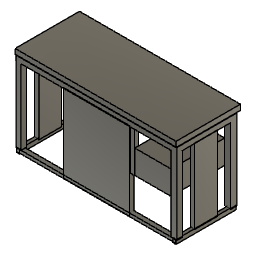
Project D2 (Autodesk Fusion 360 design; units mm, degrees)
Autodesk Fusion 360 part; units mm, degrees
sketch "Sketch1" plane through (0, 0, 0) normal (0, 1, 0) x (1, 0, 0)
  line L0 (-73.6158, -70.0302) -> (76.3842, -70.0302)
  line L1 (76.3842, -70.0302) -> (76.3842, -65.0302)
  line L2 (76.3842, -65.0302) -> (-73.6158, -65.0302)
  line L3 (-73.6158, -65.0302) -> (-73.6158, -70.0302)
  dimension "d1" = 150
  dimension "d2" = 5
  constraint horizontal L0
  constraint vertical L1
  constraint horizontal L2
  constraint vertical L3
  measures "d1" distance of L0.start L0.end
  measures "d2" distance of L0.start L2.end
extrude "Extrude1" add sketch "Sketch1" along normal blind 60 makes body 1
sketch "Sketch2" plane through (0, 0, 0) normal (0, 1, 0) x (1, 0, 0)
  line L0 (-71.4094, -65.6389) -> (74.5906, -65.6389)
  line L1 (74.5906, -65.6389) -> (74.5906, -70.6389)
  line L2 (74.5906, -70.6389) -> (-71.4094, -70.6389)
  line L3 (-71.4094, -70.6389) -> (-71.4094, -65.6389)
  dimension "d5" = 146
  dimension "d6" = 5
  constraint horizontal L0
  constraint vertical L1
  constraint horizontal L2
  constraint vertical L3
  measures "d5" distance of L0.start L0.end
  measures "d6" distance of L0.start L2.end
move_body "Move1" bodies 1 to x (1, 0, 0) y (0, 1, 0) z (0, 0, 1) at (0, 10, -40)
extrude "Extrude2" add sketch "Sketch2" along normal blind 56 separate body makes body 2
sketch "Sketch3" plane through (0, 0, 70.6389) normal (0, 0, 1) x (-1, 0, 0)
  line L0 (71.4094, 0) -> (-74.5906, 0)
  line L1 (-74.5906, 0) -> (-74.5906, -56)
  line L2 (-74.5906, -56) -> (71.4094, -56)
  line L3 (71.4094, -56) -> (71.4094, 0)
  line L4 (70, -51) -> (-70, -51)
  line L5 (-70, -51) -> (-70, -5)
  line L6 (-70, -5) -> (70, -5)
  line L7 (70, -5) -> (70, -51)
  dimension "d9" = 140
  dimension "d10" = 46
  constraint horizontal L4
  constraint vertical L5
  constraint horizontal L6
  constraint vertical L7
  measures "d9" distance of L4.start L4.end
  measures "d10" distance of L4.start L6.end
extrude "Extrude3" cut sketch "Sketch3" against normal blind 5 contours L4 L5 L6 L7 bodies 2
extrude "Extrude4" add 1 faces at (-71.4094, 18.6667, 68.9722) along direction (-1, 0, 0) blind 2 on bodies 2 bodies 2
sketch "Sketch4" plane through (0, 0, 0) normal (0, 1, 0) x (1, 0, 0)
move_body "Move2" bodies 1 to x (1, 0, 0) y (0, 1, 0) z (0, 0, 1) at (-149.7936, 0, 0)
extrude "Extrude5" add 1 faces at (-73.4094, 18.6667, 68.9722) along direction (-1, 0, 0) blind 2 on bodies 2 bodies 2
sketch "Sketch5" plane through (0, 0, 70.6389) normal (0, 0, 1) x (-1, 0, 0)
  line L0 (-70, -51) -> (-70, -5)
  line L1 (-70, -5) -> (70, -5)
  line L2 (70, -5) -> (70, -51)
  line L3 (70, -51) -> (-70, -51)
  line L4 (75.4094, 0) -> (-74.5906, 0)
  line L5 (-74.5906, 0) -> (-74.5906, -56)
  line L6 (-74.5906, -56) -> (75.4094, -56)
  line L7 (75.4094, -56) -> (75.4094, 0)
  line L8 (75.4094, -56) -> (70, -56)
  line L9 (70, -56) -> (70, -50)
  line L10 (70, -50) -> (75.4094, -50)
  line L11 (75.4094, -50) -> (75.4094, -56)
  constraint horizontal L8
  constraint vertical L9
  constraint horizontal L10
  constraint vertical L11
  constraint coincident L6.end L7.start
extrude "Extrude6" add sketch "Sketch5" along normal blind 60 contours L2 L6 L7 L8 L9 L10 L11 bodies 2
move_body "Move3" bodies 1 to x (1, 0, 0) y (0, 1, 0) z (0, 0, 1) at (-20, 0, 0)
sketch "Sketch6" plane through (0, 0, 70.6389) normal (0, 0, 1) x (-1, 0, 0)
  line L0 (70, -56) -> (70, -51)
  line L1 (70, -51) -> (-70, -51)
  line L2 (-70, -51) -> (-70, -5)
  line L3 (-70, -5) -> (70, -5)
  line L4 (70, -5) -> (70, -50)
  line L5 (70, -50) -> (75.4094, -50)
  line L6 (75.4094, -50) -> (75.4094, 0)
  line L7 (75.4094, 0) -> (-74.5906, 0)
  line L8 (-74.5906, 0) -> (-74.5906, -56)
  line L9 (-74.5906, -56) -> (70, -56)
  line L10 (-70, -56) -> (-74.4843, -56)
  line L11 (-74.4843, -56) -> (-74.4843, -51)
  line L12 (-74.4843, -51) -> (-70, -51)
  line L13 (-70, -51) -> (-70, -56)
  line L14 (-74.4843, -4.9712) -> (-70, -4.9712)
  line L15 (-70, -4.9712) -> (-70, 0)
  line L16 (-70, 0) -> (-74.4843, 0)
  line L17 (-74.4843, 0) -> (-74.4843, -4.9712)
  line L18 (70, 0) -> (75.4094, 0)
  line L19 (75.4094, 0) -> (75.4094, -5)
  line L20 (75.4094, -5) -> (70, -5)
  line L21 (70, -5) -> (70, 0)
  constraint horizontal L10
  constraint vertical L11
  constraint horizontal L12
  constraint vertical L13
  constraint coincident L9 L10.start
  constraint horizontal L14
  constraint vertical L15
  constraint horizontal L16
  constraint vertical L17
  constraint horizontal L18
  constraint vertical L19
  constraint horizontal L20
  constraint vertical L21
  constraint coincident L6 L19.end
  constraint coincident L7 L18.start
extrude "Extrude7" add sketch "Sketch6" along normal blind 70 contours L9 L10 L11 L12 L13 | L6 L7 L18 L19 L20 L21 | L7 L14 L15 L16 L17 bodies 2
extrude "Extrude8" add 1 faces at (-73.6062, 52.3333, 130.6389) along direction (0, 0, 1) blind 10 on bodies 2 bodies 2
sketch "Sketch7" plane through (0, 0, 0) normal (0, 1, 0) x (1, 0, 0)
  line L0 (-75.802, -140.9306) -> (74.198, -140.9306)
  line L1 (74.198, -140.9306) -> (74.198, -136.9306)
  line L2 (74.198, -136.9306) -> (-75.802, -136.9306)
  line L3 (-75.802, -136.9306) -> (-75.802, -140.9306)
  dimension "d23" = 150
  dimension "d24" = 4
  constraint horizontal L0
  constraint vertical L1
  constraint horizontal L2
  constraint vertical L3
  measures "d23" distance of L0.start L0.end
  measures "d24" distance of L0.start L2.end
extrude "Extrude9" add sketch "Sketch7" against normal blind 5 bodies 2
delete_face "DeleteFace1" 1 faces at (-23.868, -3.3333, 136.9306) on bodies 2
sketch "Sketch8" plane through (0, 0, 0) normal (0, 1, 0) x (1, 0, 0)
  line L0 (74, -147) -> (-74, -147)
  line L1 (-74, -147) -> (-74, -144)
  line L2 (-74, -144) -> (74, -144)
  line L3 (74, -144) -> (74, -147)
  dimension "d27" = 148
  dimension "d28" = 3
  constraint horizontal L0
  constraint vertical L1
  constraint horizontal L2
  constraint vertical L3
  measures "d27" distance of L0.start L0.end
  measures "d28" distance of L0.start L2.end
extrude "Extrude10" add sketch "Sketch8" along normal blind 4 separate body makes body 3
move_body "Move4" bodies 3 to x (1, 0, 0) y (0, 1, 0) z (0, 0, 1) at (0, 0, -3)
sketch "Sketch9" plane through (0, 0, 0) normal (1, 0, 0) x (0, 1, 0)
  line L0 (55.6729, 149.8662) -> (-0.3271, 149.8662)
  line L1 (-0.3271, 149.8662) -> (-0.3271, 145.8662)
  line L2 (-0.3271, 145.8662) -> (55.6729, 145.8662)
  line L3 (55.6729, 145.8662) -> (55.6729, 149.8662)
  dimension "d31" = 56
  dimension "d32" = 4
  constraint horizontal L0
  constraint vertical L1
  constraint horizontal L2
  constraint vertical L3
  measures "d31" distance of L0.start L0.end
  measures "d32" distance of L0.start L2.end
extrude "Extrude11" add sketch "Sketch9" along normal blind 3 separate body makes body 4
copy_body "CopyPasteBodies1" bodies 4 makes body 5
move_body "Move5" bodies 4 to x (1, 0, 0) y (0, 1, 0) z (0, 0, 1) at (-75, 0, 0)
move_body "Move6" bodies 5 to x (1, 0, 0) y (0, 1, 0) z (0, 0, 1) at (65, 0, 0)
move_face "MoveFace1" by (0, 0, -5) 1 faces at (-74, -0.3271, 148.5329) on bodies 4
move_body "Move7" bodies 4 to x (1, 0, 0) y (0, 1, 0) z (0, 0, 1) at (0, 0, -6)
move_body "Move8" bodies 3 to x (1, 0, 0) y (0, 1, 0) z (0, 0, 1) at (0, 0, -0.5)
move_body "Move9" bodies 5 to x (1, 0, 0) y (0, 1, 0) z (0, 0, 1) at (6, 0, -6)
sketch "Sketch10" plane through (0, 0, 0) normal (1, 0, 0) x (0, 1, 0)
  line L0 (38.1353, 140.4683) -> (16.8639, 140.4683)
  line L1 (16.8639, 140.4683) -> (16.8639, 70.33)
  line L2 (16.8639, 70.33) -> (38.1353, 70.33)
  line L3 (38.1353, 70.33) -> (38.1353, 140.4683)
  constraint horizontal L0
  constraint vertical L1
  constraint horizontal L2
  constraint vertical L3
extrude "Extrude12" add sketch "Sketch10" along normal blind 4 separate body makes body 6
copy_body "CopyPasteBodies2" bodies 6 makes body 7
move_body "Move10" bodies 7 to x (1, 0, 0) y (0, 1, 0) z (0, 0, 1) at (-75, 0, 0)
move_body "Move11" bodies 6 to x (1, 0, 0) y (0, 1, 0) z (0, 0, 1) at (70, 0, 0)
sketch "Sketch11" plane through (0, 0, 0) normal (0, 1, 0) x (1, 0, 0)
  line L0 (-31.433, -63.1947) -> (30, -63.1947)
  line L1 (30, -63.1947) -> (30, 10)
  line L2 (30, 10) -> (-31.433, 10)
  line L3 (-31.433, 10) -> (-31.433, -63.1947)
  dimension "d37" = 61.433
  constraint horizontal L0
  constraint vertical L1
  constraint horizontal L2
  constraint vertical L3
  measures "d37" distance of L0.start L0.end
extrude "Extrude13" add sketch "Sketch11" along normal blind 4 separate body makes body 8
move_body "Move12" bodies 8 to x (1, 0, 0) y (0, 1, 0) z (0, 0, 1) at (0, 0, 80)
sketch "Sketch12" plane through (0, 0, 0) normal (0, 1, 0) x (1, 0, 0)
  line L0 (-69.4048, -85.616) -> (-35.6434, -85.616)
  line L1 (-35.6434, -85.616) -> (-35.6434, -107.7355)
  line L2 (-35.6434, -107.7355) -> (-69.4048, -107.7355)
  line L3 (-69.4048, -107.7355) -> (-69.4048, -85.616)
  dimension "d40" = 33.7613
  constraint horizontal L0
  constraint vertical L1
  constraint horizontal L2
  constraint vertical L3
  measures "d40" distance of L0.start L0.end
extrude "Extrude14" add sketch "Sketch12" along normal blind 50 separate body makes body 9
move_face "MoveFace2" by (-2, 0, 0) 1 faces at (-46.8972, 50, 100.3623) on bodies 9
move_body "Move13" bodies 9 to x (1, 0, 0) y (0, 1, 0) z (0, 0, 1) at (-0.6, 0, 0)
sketch "Sketch13" plane through (0, 0, 0) normal (0, 1, 0) x (1, 0, 0)
  line L0 (-35.8945, -108.0202) -> (-32.1443, -108.0202)
  line L1 (-32.1443, -108.0202) -> (-32.1443, -70.7152)
  line L2 (-32.1443, -70.7152) -> (-35.8945, -70.7152)
  line L3 (-35.8945, -70.7152) -> (-35.8945, -108.0202)
  dimension "d43" = 3.7502
  constraint horizontal L0
  constraint vertical L1
  constraint horizontal L2
  constraint vertical L3
  measures "d43" distance of L0.start L0.end
extrude "Extrude15" add sketch "Sketch13" along normal blind 4 separate body makes body 10
copy_body "CopyPasteBodies3" bodies 10 makes body 11
move_body "Move14" bodies 11 to x (1, 0, 0) y (0, 1, 0) z (0, 0, 1) at (0, 1000, 0)
move_body "Move15" bodies 1 to x (1, 0, 0) y (0, 1, 0) z (0, 0, 1) at (190, 0, -100)
move_body "Move16" bodies 7 10 5 6 11 3 4 2 8 9 to x (-1, 0, 0) y (0, 1, 0) z (0, 0, -1) at (21.9612, 0, 76.0403)
move_body "Move17" bodies 1 to x (1, 0, 0) y (0, 1, 0) z (0, 0, 1) at (0, 0, 85)
move_body "Move18" bodies 1 to x (1, 0, 0) y (0, 1, 0) z (0, 0, 1) at (0, -10, 0)
sketch "Sketch14" plane through (0, 0, 0) normal (0, 1, 0) x (1, 0, 0)
sketch "Sketch15" plane through (0, 0, 0) normal (0, 0, 1) x (1, 0, 0)
move_body "Move19" bodies 11 to x (1, 0, 0) y (0, 1, 0) z (0, 0, 1) at (0, -950, 0)
named bodies: "Top", "Frame"
